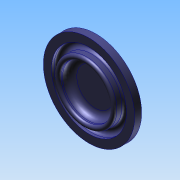
# Autodesk Inventor part: BFA 30 25 10 530043 Rollmembran mittel
Saved by Autodesk Inventor 2015 (Build 190159000, 159)
## iProperties
Category: PARTsolutions
Company: SIMRIT
Created: 2015-06-19
Part Number: BFA 30 25 10 530043 Rollmembran mittel
Catalog Web Link: www.cadenas.de
Description: BFA-Rolling diaphragms
Vendor: SIMRIT
Document SubType Name: Modeling
Designer: PARTuser1
Manufacturer: SIMRIT
Mass: 3.28845 g
Surface Area: 52.3808 cm^2
Volume: 2.63076 cm^3
Density: 1.25 g/cm^3
Material: Gummi, Silikon
Appearance: PSOLRGB-127-127-255
PSOL_IDENT_0: {$CADENAS_DATA\23d-libs\simrit\spezialdichtungsprodukte\membranen\rollmembranen\bfa\bfa.prj},199 {VT
PSOL_IDENT_1: YP=3D},{NB=BFA 30 25 10 530043 Rollmembran mittel},{LINA=BFA 30 25 10 530043},{NN=BFA},{DATE=13.03.2
PSOL_IDENT_2: 015 08:01:04},{GEOMDATE=05.12.2013 13:36:00},{VERSION=},{LINEID=60},{LINESUBID=-1},{WBVAR=AUS}  {NB=
PSOL_IDENT_3: BFA 30 25 10 530043 Rollmembran mittel},{LINA=BFA 30 25 10 530043},{KT=DUMMY},{IDNR=},{ARTIKELNR=530
PSOL_IDENT_4: 043},{BF=BFA},{WS=50 NBR 253},{AUS=Rollmembran mittel},{DC=30},{DK=25},{H=10},{W=0.45},{VERS=1.000},
PSOL_IDENT_5: {DN=45.000},{RK=3.500},{HI=3.000},{HG=3.450},{WG=4.000},{SB2=147.427},{SA=2.000},{YDATUM21=150.000},
PSOL_IDENT_6: {RI=1.750},{SA1=2.000},{SB1=2.000},{XX=2.450}
SUPPLIER: SIMRIT
ARTICLENO: BFA 30 25 10 530043 Rollmembran mittel
BOMINFO: BFA 30 25 10 530043
CREATOR: CADENAS GmbH
Title: BFA 30 25 10 530043
Author: Cadenas PARTsolutions
Comments: Rolling diaphragms
Autodesk Inventor part; units mm, degrees
ref_plane "YZ Plane" through (0, 0, 0) normal (1, 0, 0) x (0, 1, 0)
ref_plane "XZ Plane" through (0, 0, 0) normal (0, 1, 0) x (-1, 0, 0)
ref_plane "XY Plane" through (0, 0, 0) normal (0, 0, 1) x (1, 0, 0)
sketch "Skizze4" plane through (0, 0, 0) normal (0, 1, 0) x (-1, 0, 0)
  point P0 (0, 0)
  point P1 (0, 0)
  constraints: 1 coincident
sketch "Sketch_2" plane through (0, 0, 0) normal (0, 0, 1) x (1, 0, 0)
  line L0 (0, -0.225) -> (0, 0.225)
  line L1 (0, 0.225) -> (9, 0.225)
  arc A0 (12.95, -3.725) -> (9, 0.225) centre (9, -3.725) ccw
  line L2 (12.95, -3.725) -> (12.95, -4.425)
  arc A1 (12.95, -4.425) -> (14.55, -4.425) centre (13.75, -4.425) ccw
  line L3 (14.55, -4.425) -> (14.55, -1.975)
  arc A2 (16.75, 0.225) -> (14.55, -1.975) centre (16.75, -1.975) ccw
  line L4 (16.75, 0.225) -> (22.5, 0.225)
  line L5 (22.5, 0.225) -> (22.5, -3.225)
  line L6 (22.5, -3.225) -> (18.5, -3.225)
  line L7 (18.5, -3.225) -> (18.5, -1.975)
  arc A3 (18.5, -1.975) -> (15, -1.975) centre (16.75, -1.975) ccw
  line L8 (15, -1.975) -> (15, -4.425)
  arc A4 (12.5, -4.425) -> (15, -4.425) centre (13.75, -4.425) ccw
  line L9 (12.5, -4.425) -> (12.5, -3.725)
  arc A5 (12.5, -3.725) -> (9, -0.225) centre (9, -3.725) ccw
  line L10 (9, -0.225) -> (0, -0.225)
  line L11 (0, -0.225) -> (0, 0.225)
  point P0 (0, 0)
  point P1 (0, 0)
  point P2 (0, 0)
  dimension "d1" = 4
  dimension "d2" = 3.45
  dimension "d3" = 3.5
  dimension "d4" = 1.6
  dimension "d5" = 9
  dimension "d6" = 0.45
  dimension "d7" = 9
  dimension "d8" = 3.5
  dimension "d9" = 5.75
  dimension "d10" = 1.25
  dimension "d11" = 2.2
  dimension "d12" = 22.5
  dimension "d13" = 16.75
  dimension "d14" = 18.5
  dimension "d22" = 0.45
  dimension "d25" = 0.45
  dimension "d26" = 0.45
  dimension "d28" = 0.7
  dimension "d29" = 2.45
  dimension "d30" = 3
  constraints: 24 end point, 12 point on circle, 12 tangent, 6 centre point, 3 horizontal, 2 coincident, 2 midpoint, 2 vertical, 1 vertical alignment
  measures "d1" distance of L5.end L6.end
  measures "d2" distance of L4.end L5.end
  measures "d3" distance between parallel lines of L8 L7
  measures "d4" distance between parallel lines of L2 L3
  measures "d5" distance of L1.start L1.end
  measures "d6" distance of L0.start L0.end
  measures "d7" distance of L10.start L10.end
  measures "d8" radius of A5
  measures "d9" distance of L4.start L4.end
  measures "d10" distance of L6.end L7.end
  measures "d11" distance from line of L4 L7.end
  measures "d12" distance between parallel lines of L0 L5
  measures "d13" distance from line of L0 L4.start
  measures "d14" distance between parallel lines of L0 L7
  measures "d22" radial gap between concentric circles of A0 A5
  measures "d25" distance between parallel lines of L9 L2
  measures "d26" radial gap between concentric circles of A4 A1
  measures "d28" vertical distance of A1.centre A0.centre
  measures "d29" vertical distance of A2.centre A1.centre
  measures "d30" horizontal distance of A1.centre A2.centre
revolve "Revolution1" add sketch "Sketch_2" angle 360 about axis through (0, -0.225, 0) along (0, -1, 0)
body "Solid1"
